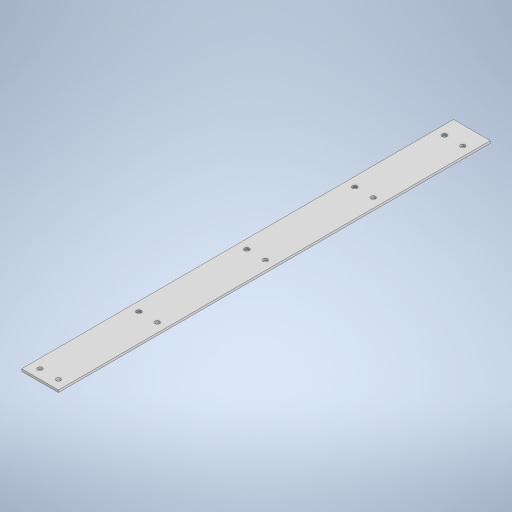
# Autodesk Inventor part: Plate2inx47in
Saved by Autodesk Inventor 2023 (Build 270158030, 158C)
## iProperties
Created: 2023-02-14
Part Number: Plate2inx47in
Material: Generic
Document SubType Name: Modeling
Designer: jeremyy
Density: 1 g/cm^3
Appearance: Default
Author: jeremyy
Autodesk Inventor part; units mm, degrees
ref_plane "YZ Plane" through (0, 0, 0) normal (1, 0, 0) x (0, 1, 0)
ref_plane "XZ Plane" through (0, 0, 0) normal (0, 1, 0) x (-1, 0, 0)
ref_plane "XY Plane" through (0, 0, 0) normal (0, 0, 1) x (1, 0, 0)
sketch "Sketch1" plane through (0, 0, 0) normal (0, 1, 0) x (-1, 0, 0)
  line L0 (0, 0) -> (50.8, 0)
  line L1 (50.8, 0) -> (50.8, -596.9)
  line L2 (50.8, -596.9) -> (0, -596.9)
  line L3 (0, -596.9) -> (0, 0)
  circle A0 centre (38.1, -12.7) radius 3.175
  line L4 (25.4, 0) -> (25.4, -12.7)
  circle A1 centre (38.1, -571.5) radius 3.175
  circle A2 centre (38.1, -298.45) radius 3.175
  circle A3 centre (12.7, -571.5) radius 3.175
  circle A4 centre (12.7, -298.45) radius 3.175
  circle A5 centre (12.7, -12.7) radius 3.175
  circle A6 centre (38.1, -149.225) radius 3.175
  line L5 (0, -298.45) -> (4.0649, -298.45)
  circle A7 centre (12.7, -149.225) radius 3.175
  circle A8 centre (38.1, -447.675) radius 3.175
  circle A9 centre (12.7, -447.675) radius 3.175
  dimension "d0" = 50.8
  dimension "d1" = 596.9
  dimension "d4" = 6.35
  dimension "d5" = 12.7
  dimension "d6" = 12.7
  dimension "d11" = 6.35
  dimension "d12" = 298.45
  dimension "d13" = 6.35
  dimension "d14" = 149.225
  constraints: 12 end point, 10 centre point, 6 symmetric about line, 2 horizontal, 2 midpoint, 2 parallel, 1 coincident, 1 perpendicular, 1 vertical, 5 other
  measures "d0" distance of L1.end L2.end
  measures "d1" distance of L0.end L1.end
  measures "d4" diameter of A0
  measures "d5" distance from line of L1 A0.centre
  measures "d6" distance from line of L0 A0.centre
  measures "d11" diameter of A5
  measures "d12" distance from line of L0 A2.centre
  measures "d13" diameter of A6
  measures "d14" distance from line of L0 A6.centre
extrude "Extrusion1" add sketch "Sketch1" along normal blind 3.175
body "Solid1"
